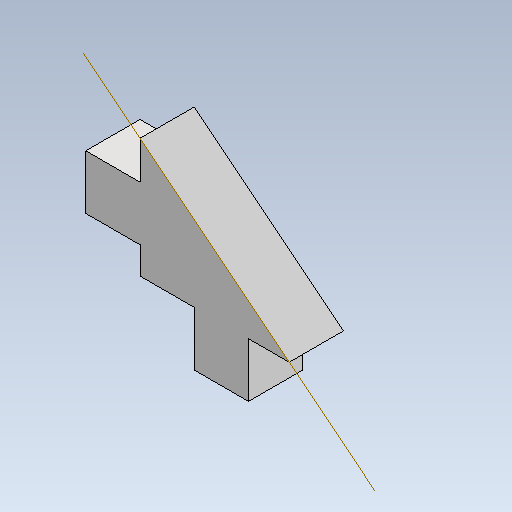
# Autodesk Inventor part: camera-bracket-rib
Saved by Autodesk Inventor 2025 (Build 290162000, 162)
## iProperties
Created: 2025-08-26
Part Number: camera-bracket-rib
Material: Generic
Document SubType Name: Modeling
Designer: HP
Density: 1 g/cm^3
Appearance: Default
Author: HP
Autodesk Inventor part; units mm, degrees
ref_plane "YZ Plane" through (0, 0, 0) normal (1, 0, 0) x (0, 1, 0)
ref_plane "XZ Plane" through (0, 0, 0) normal (0, 1, 0) x (-1, 0, 0)
ref_plane "XY Plane" through (0, 0, 0) normal (0, 0, 1) x (1, 0, 0)
sketch "Sketch1" plane through (0, 0, 0) normal (0, 0, 1) x (1, 0, 0)
  line L0 (-12.5, -10) -> (12.5, -10)
  line L1 (12.5, -10) -> (12.5, 10) construction
  line L2 (12.5, 10) -> (-12.5, 10) construction
  line L3 (-12.5, 10) -> (-12.5, -10)
  line L4 (-12.5, -10) -> (12.5, 10) construction
  line L5 (12.5, -10) -> (-12.5, 10)
  line L6 (-12.5, -2.5) -> (-7.5, -2.5)
  line L7 (-7.5, -2.5) -> (-7.5, 2.5) construction
  line L8 (-7.5, 2.5) -> (-12.5, 2.5)
  line L9 (-12.5, 2.5) -> (-12.5, -2.5)
  line L10 (-12.5, -2.5) -> (-7.5, 2.5) construction
  line L11 (-7.5, -2.5) -> (-12.5, 2.5) construction
  line L12 (-7.5, -2.5) -> (-7.5, -10)
  line L13 (-7.5, 2.5) -> (-7.5, 6)
  line L14 (-2.5, -10) -> (2.5, -10)
  line L15 (2.5, -10) -> (2.5, -5)
  line L16 (2.5, -5) -> (-2.5, -5) construction
  line L17 (-2.5, -5) -> (-2.5, -10)
  line L18 (-2.5, -10) -> (2.5, -5) construction
  line L19 (2.5, -10) -> (-2.5, -5) construction
  line L20 (-2.5, -5) -> (-7.5, -5)
  line L21 (2.5, -5) -> (6.25, -5)
  point P0 (0, 0)
  point P1 (-10, 0)
  point P2 (0, 0)
  point P3 (0, -7.5)
  point P4 (2.5, -10)
  dimension "d0" = 20
  dimension "d1" = 25
  dimension "d2" = 5
  dimension "d3" = 5
  dimension "d4" = 10
  dimension "d5" = 5
  dimension "d6" = 5
  dimension "d7" = 12.5
  constraints: 44 end point, 6 midpoint, 6 parallel, 6 point on line, 5 perpendicular, 3 horizontal, 2 collinear, 1 coincident
  measures "d0" distance between parallel lines of L2 L0
  measures "d1" distance between parallel lines of L1 L3
  measures "d2" distance between parallel lines of L7 L9
  measures "d3" distance between parallel lines of L6 L8
  measures "d4" distance from line of L0 point (-10, 0)
  measures "d5" distance of L16.end L15.end
  measures "d6" distance between parallel lines of L14 L16
  measures "d7" distance from line of L3 point (0, -7.5)
extrude "Extrusion1" add sketch "Sketch1" along normal blind 5 contours L3 L8 L13 L5 L21 L15 L0 L17 L20 L12 L6
equation "\"d5\" = d3"
equation "\"d6\" = d2"
body "Solid1"
